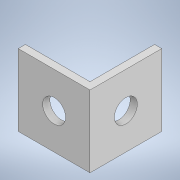
# Autodesk Inventor part: No Thrd Right Support Farnell1466881
Saved by Autodesk Inventor 2021 (Build 250183000, 183)
## iProperties
Created: 2020-08-05
Part Number: No Thrd Right Support Farnell1466881
Material: Generic
Document SubType Name: Modeling
Designer: jgray
Density: 1 g/cm^3
Appearance: Default
Author: jgray
Autodesk Inventor part; units mm, degrees
ref_plane "YZ Plane" through (0, 0, 0) normal (1, 0, 0) x (0, 1, 0)
ref_plane "XZ Plane" through (0, 0, 0) normal (0, 1, 0) x (-1, 0, 0)
ref_plane "XY Plane" through (0, 0, 0) normal (0, 0, 1) x (1, 0, 0)
sketch "Sketch1" plane through (0, 0, 0) normal (0, 1, 0) x (-1, 0, 0)
  line L0 (0.8918, 0) -> (0, 0)
  line L1 (0, 0) -> (0, -10)
  line L2 (0, 0) -> (10, 0)
  line L3 (10, 0) -> (10, -1)
  line L4 (10, -1) -> (1, -1)
  line L5 (1, -1) -> (1, -10)
  line L6 (1, -10) -> (0, -10)
  dimension "d1" = 10
  dimension "d2" = 10
  dimension "d3" = 1
  dimension "d4" = 9
  dimension "d5" = 9
  constraints: 14 end point, 5 perpendicular, 1 horizontal
  measures "d1" distance of L0.end L1.end
  measures "d2" distance of L0.end L2.end
  measures "d3" distance of L2.end L3.end
  measures "d4" distance of L3.end L4.end
  measures "d5" distance of L4.end L5.end
extrude "Extrusion1" add sketch "Sketch1" along normal blind 10
sketch "Sketch2" plane through (-10, 0, 0) normal (0, 0, 1) x (1, 0, 0)
  line L0 (-6.0649, 5) -> (16.1228, 5) construction
  line L1 (5, 14.125) -> (5, -1.5964) construction
  line L2 (0, 10) -> (10, 10) construction
  line L3 (10, 0) -> (10, 10) construction
  point P0 (5, 10)
  point P1 (10, 5)
  point P2 (5, 5)
  constraints: 4 end point, 4 point on line, 2 midpoint, 1 horizontal, 1 vertical
hole "Hole1" at (-5, 5, 0) direction (0, 0, -1) diameter 3.2 end through all
sketch "Sketch3" plane through (0, 0, 0) normal (1, 0, 0) x (0, 0, -1)
  line L0 (5, 14.0037) -> (5, -2.6876)
  line L1 (-5.0316, 5) -> (14.0442, 5)
  line L2 (0, 10) -> (10, 10) projected
  line L3 (10, 0) -> (10, 10) projected
  point P0 (0, 0)
  point P1 (5, 10)
  point P2 (10, 5)
  point P3 (5, 5)
  constraints: 4 end point, 4 point on line, 2 midpoint, 1 horizontal, 1 vertical
hole "Hole2" at (0, 5, -5) direction (-1, 0, 0) diameter 3.2 end through all
body "Solid1"
